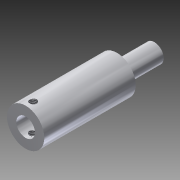
# Autodesk Inventor part: Extender
Saved by Autodesk Inventor 2015 (Build 190159000, 159)
## iProperties
Created: 2015-01-06
Part Number: Extender
Material: Aluminum 6061
Document SubType Name: Modeling
Designer: ice
Mass: 1.90852 g
Surface Area: 13.1319 cm^2
Volume: 1.90852 cm^3
Density: 2.7 g/cm^3
Appearance: Aluminum - Flat
Author: ice
Autodesk Inventor part; units mm, degrees
ref_plane "YZ Plane" through (0, 0, 0) normal (1, 0, 0) x (0, 1, 0)
ref_plane "XZ Plane" through (0, 0, 0) normal (0, 1, 0) x (-1, 0, 0)
sketch "Sketch1" plane through (0, 0, 0) normal (1, 0, 0) x (0, 1, 0)
  line L0 (0, 2.5) -> (-4, 2.5)
  line L1 (-4, 5) -> (2, 5)
  line L2 (30, 2.5) -> (20, 2.5)
  line L3 (20, 2.5) -> (20, 5)
  line L4 (20, 5) -> (2, 5)
  line L5 (30, 1) -> (0, 1)
  line L6 (0, 0) -> (31.6248, 0)
  arc A0 (30, 2.2) -> (30, 1.3) centre (30, 1.75) ccw
  line L7 (30, 1.25) -> (30, 1.3)
  line L8 (30, 2.2) -> (30, 2.25)
  line L9 (30, 1) -> (30, 1.3)
  line L10 (30, 2.2) -> (30, 2.5)
  arc A1 (0, 1.3) -> (0, 2.2) centre (0, 1.75) ccw
  line L11 (0, 1) -> (0, 1.3)
  line L12 (0, 2.2) -> (0, 2.5)
  line L13 (0, 1.25) -> (0, 1.3)
  line L14 (0, 2.2) -> (0, 2.25)
  line L15 (-4, 5) -> (0, 5)
  line L16 (-4, 5) -> (-4.5, 5)
  line L17 (-4.5, 5) -> (-4.5, 2.5)
  line L18 (-4.5, 2.5) -> (-4, 2.5)
  dimension "d0" = 2.5
  dimension "d2" = 2.5
  dimension "d6" = 10
  dimension "d7" = 2.5
  dimension "d32" = 0.9
  dimension "d33" = 0.3
  dimension "d34" = 1.75
  dimension "d35" = 0.9
  dimension "d36" = 2.5
  dimension "d37" = 1.75
  dimension "d39" = 20
  dimension "d41" = 4.5
  constraints: 38 end point, 9 perpendicular, 5 point on line, 4 point on circle, 4 vertical, 2 centre point, 2 horizontal
  measures "d0" distance of L6.start L0.start
  measures "d2" distance of L0.end L1.start
  measures "d6" distance of L2.start L2.end
  measures "d7" distance of L2.end L3.end
  measures "d32" distance of L12.start L11.end
  measures "d33" distance of L0.start L12.start
  measures "d34" distance of L6.start A1.centre
  measures "d35" distance of L8.start L7.end
  measures "d36" distance from line of L6 L2.start
  measures "d37" distance from line of L6 A0.centre
  measures "d39" distance of L3.end L15.end
  measures "d41" distance of L16.end L15.end
revolve "Revolution1" add sketch "Sketch1" angle 360 about axis through (0, 0, 0) along (0, 1, 0)
ref_plane "Work Plane2" through (0, 0, 5) normal (0, 0, 1) x (1, 0, 0)
sketch "Sketch5" plane through (0, 0, 5) normal (0, 0, 1) x (1, 0, 0)
  line L0 (5, -4) -> (-5, -4) projected
  line L1 (0, -1) -> (0, -2.5)
  dimension "d44" = 1.5
  constraints: 2 end point, 1 vertical
  measures "d44" distance of L1.start L1.end
hole "Hole1" at (0, -2.5, 5) direction (0, 0, -1) diameter 1.9 end through all
thread "Thread3" size "M2x0.4" class "6H" standard "ANSI Metric M Profile" full length
thread "Thread4" size "M2x0.4" class "6H" standard "ANSI Metric M Profile" full length
body "Solid1"
